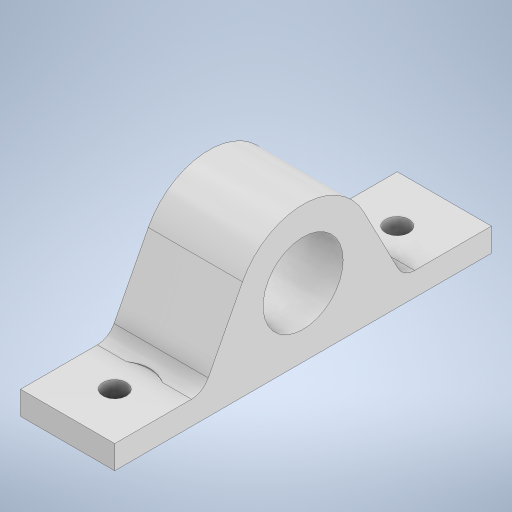
# Autodesk Inventor part: base_axis_8mm_2020
Saved by Autodesk Inventor 2024 (Build 280153000, 153)
## iProperties
Created: 2025-12-25
Part Number: base_axis_8mm_2020
Material: PET Plastic
Document SubType Name: Modeling
Designer: schar
Density: 1.541 g/cm^3
Appearance: Polycarbonate - Clear
Author: schar
Autodesk Inventor part; units mm, degrees
ref_plane "YZ Plane" through (0, 0, 0) normal (1, 0, 0) x (0, 1, 0)
ref_plane "XZ Plane" through (0, 0, 0) normal (0, 1, 0) x (-1, 0, 0)
ref_plane "XY Plane" through (0, 0, 0) normal (0, 0, 1) x (1, 0, 0)
sketch "Sketch1" plane through (0, 0, 0) normal (1, 0, 0) x (0, 1, 0)
  line L0 (0, 0) -> (5, 0)
  line L1 (5, 0) -> (5, -40)
  line L2 (5, -40) -> (0, -40)
  line L3 (0, -40) -> (0, 0)
  line L4 (5, -20) -> (10.5, -20)
  circle A0 centre (10.5, -20) radius 4
  line L5 (10.5, -16) -> (5, -16)
  line L6 (10.5, -24) -> (5, -24)
  circle A1 centre (10.5, -20) radius 5.5
  line L7 (14.277, -16.0019) -> (5, -7.2379)
  line L8 (14.2701, -24.0045) -> (5, -32.7321)
  dimension "d0" = 5
  dimension "d1" = 40
  dimension "d2" = 5.5
  dimension "d3" = 8
  constraints: 18 end point, 5 point on circle, 4 point on line, 4 tangent, 3 horizontal, 2 centre point, 2 coincident, 2 parallel, 2 perpendicular, 1 midpoint
  measures "d0" distance of L1.end L2.end
  measures "d1" distance of L0.end L1.end
  measures "d2" distance of L4.start L4.end
  measures "d3" diameter of A0
extrude "Extrusion1" add sketch "Sketch1" along normal blind 20 contours L0 L1 L2 L3 | L7 A1 L5 L1 | L5 A1 L1 | A1 L6 A0 L5 | L1 L6 A1 L8 | A1 L6 L1 | A1 L5 A0 L4 | L4 A0 L6 A1
sketch "Sketch2" plane through (0, 0, -40) normal (0, 0, -1) x (-1, 0, 0)
  line L0 (0, 5) -> (-20, 5) projected
  line L1 (-20, 5) -> (0, 5)
  line L2 (0, 5) -> (0, 0)
  line L3 (0, 0) -> (-20, 0)
  line L4 (-20, 0) -> (-20, 5)
  constraints: 8 end point, 2 parallel, 1 horizontal, 1 perpendicular
extrude "Extrusion2" add sketch "Sketch2" along normal blind 20
sketch "Sketch3" plane through (0, 0, 0) normal (0, 0, 1) x (1, 0, 0)
  line L0 (0, 5) -> (20, 5) projected
  line L1 (20, 5) -> (20, 0) projected
  line L2 (0, 5) -> (20, 5)
  line L3 (20, 5) -> (20, 0)
  line L4 (20, 0) -> (0, 0)
  line L5 (0, 0) -> (0, 5)
  constraints: 8 end point, 2 parallel, 1 horizontal, 1 perpendicular
extrude "Extrusion3" add sketch "Sketch3" along normal blind 20
fillet "Fillet1" radius 4 2 edges at (10, 5, -32.7321) (10, 5, -7.2379)
sketch "Sketch4" plane through (0, 5, 20) normal (0, 1, 0) x (1, 0, 0)
  line L0 (0, 80) -> (0, 0) projected
  line L1 (0, 0) -> (10, 0)
  line L2 (0, 0) -> (20, 0) projected
  line L3 (10, 0) -> (10, 10)
  circle A0 centre (10, 10) radius 2.5
  line L4 (0, 80) -> (10, 80)
  line L5 (0, 80) -> (20, 80) projected
  line L6 (10, 80) -> (10, 70)
  circle A1 centre (10, 70) radius 2.5
  point P0 (0, 20)
  dimension "d11" = 10
  dimension "d12" = 10
  dimension "d13" = 5
  dimension "d14" = 10
  dimension "d15" = 5
  constraints: 8 end point, 2 centre point, 2 coincident, 2 midpoint, 2 perpendicular
  measures "d11" distance of L0.end L1.end
  measures "d12" distance of L1.end L3.end
  measures "d13" diameter of A0
  measures "d14" distance of L4.end L6.end
  measures "d15" diameter of A1
extrude "Extrusion4" cut sketch "Sketch4" against normal blind 20
sketch "Sketch5" plane through (20, 0, 0) normal (1, 0, 0) x (0, 0, -1)
  circle A0 centre (20, 10.5) radius 4 projected
  circle A1 centre (20, 10.5) radius 7
  line L0 (16, 16.2446) -> (0, 5)
  line L1 (5.5141, 5) -> (-20, 5) projected
  line L2 (34.46, 5) -> (60, 5) projected
  line L3 (20, 17.5) -> (20, 10.5)
  line L4 (24, 16.2446) -> (40, 5)
  line L5 (40, 5) -> (24.3301, 5)
  line L6 (0, 5) -> (15.6699, 5)
  point P0 (0, 0)
  point P1 (40, 5)
  dimension "d18" = 14
  constraints: 10 end point, 4 point on circle, 2 point on line, 2 symmetric about line, 1 centre point, 1 coincident, 1 horizontal, 1 vertical
  measures "d18" diameter of A1
extrude "Extrusion5" add sketch "Sketch5" against normal blind 20
fillet "Fillet2" radius 4 2 edges at (10, 5, -40) (10, 5, 0)
sketch "Sketch6" plane through (0, 0, 0) normal (-1, 0, 0) x (0, 0, 1)
  circle A0 centre (-20, 10.5) radius 4 projected
  line L0 (-20, 10.5) -> (-20, 14.5)
  circle A1 centre (-20, 14.5) radius 11
  circle A2 centre (-20, 14.5) radius 14.5
  arc A3 (-41.265, 5) -> (-38.965, 5.7274) centre (-41.265, 9) ccw projected
  line L1 (-41.265, 5) -> (-32.8706, 21.1782)
  line L2 (1.265, 5) -> (20, 5) projected
  line L3 (1.265, 5) -> (-7.1294, 21.1782)
  line L4 (-41.265, 5) -> (-23.6138, 0.4575)
  arc A4 (-1.035, 5.7274) -> (1.265, 5) centre (1.265, 9) ccw projected
  line L5 (-16.3862, 0.4575) -> (1.265, 5)
  point P0 (0, 0)
  dimension "d23" = 4
  dimension "d24" = 22
  constraints: 10 end point, 4 point on circle, 3 tangent, 2 centre point, 2 coincident, 1 vertical
  measures "d23" distance of L0.start L0.end
  measures "d24" diameter of A1
extrude "Extrusion6" add sketch "Sketch6" against normal blind 20 contours A2 | A2 L3 L5 | A2 L4 L1
sketch "Sketch7" plane through (0, 0, 0) normal (-1, 0, 0) x (0, 0, 1)
  circle A0 centre (-20, 10.5) radius 4 projected
  circle A1 centre (-20, 14.5) radius 11
  point P0 (0, 0)
  constraints: 1 centre point, 1 vertical alignment, 1 other
extrude "Extrusion7" cut sketch "Sketch7" against normal blind 20
fillet "Fillet3" radius 4 2 edges at (10, 5, -41.265) (10, 5, 1.265)
sketch "Sketch8" plane through (0, 5, 20) normal (0, 1, 0) x (1, 0, 0)
  circle A0 centre (10, 10) radius 2.5 projected
  circle A1 centre (10, 10) radius 7.4
  circle A2 centre (10, 70) radius 2.5 projected
  circle A3 centre (10, 70) radius 7.4
  point P0 (0, 20)
  dimension "d30" = 14.8
  dimension "d31" = 14.8
  constraints: 2 centre point, 2 coincident
  measures "d30" diameter of A1
  measures "d31" diameter of A3
extrude "Extrusion8" cut sketch "Sketch8" along normal blind 10
sketch "Sketch9" plane through (20, 0, 0) normal (1, 0, 0) x (0, 0, -1)
  circle A0 centre (20, 14.5) radius 11 projected
  circle A1 centre (20, 14.5) radius 11
  circle A2 centre (20, 14.5) radius 8.5
  point P0 (0, 0)
  dimension "d34" = 17
  constraints: 2 centre point, 2 coincident
  measures "d34" diameter of A2
extrude "Extrusion9" add sketch "Sketch9" against normal blind 12
body "Solid1"
